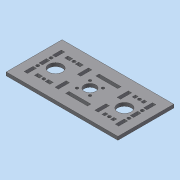
# Autodesk Inventor part: Camera-Holder_Front
Saved by Autodesk Inventor 2016 SP1 (Build 200210100, 210)
## iProperties
Created: 2016-01-24
Part Number: Camera-Holder_Front
Material: Generic
Document SubType Name: Modeling
Designer: Mohamed A.
Density: 1 g/cm^3
Appearance: Default
Author: Mohamed A.
Autodesk Inventor part; units mm, degrees
ref_plane "YZ Plane" through (0, 0, 0) normal (1, 0, 0) x (0, 1, 0)
ref_plane "XZ Plane" through (0, 0, 0) normal (0, 1, 0) x (-1, 0, 0)
ref_plane "XY Plane" through (0, 0, 0) normal (0, 0, 1) x (1, 0, 0)
sketch "Sketch1" plane through (0, 0, 0) normal (0, 0, 1) x (1, 0, 0)
  circle A0 centre (-5.816, 5.816) radius 1.25
  circle A1 centre (5.816, 5.816) radius 1.25
  circle A2 centre (5.816, -5.816) radius 1.25
  circle A3 centre (-5.816, -5.816) radius 1.25
  circle A4 centre (0, 0) radius 11
  circle A5 centre (0, 0) radius 5.125
  circle A6 centre (30.8333, 0) radius 6.096
  circle A7 centre (-30.8333, 0) radius 6.096
  line L0 (30.8333, 0) -> (-30.8333, 0) construction
  line L1 (-60, 25) -> (60, 25)
  line L2 (60, 25) -> (60, -25)
  line L3 (60, -25) -> (-60, -25)
  line L4 (-60, -25) -> (-60, 25)
  line L5 (0, 25) -> (0, -25) construction
  point P0 (0, 0)
  dimension "d9" = 2.5
  dimension "d10" = 2.5
  dimension "d11" = 2.5
  dimension "d12" = 2.5
  dimension "d33" = 120
  dimension "d34" = 50
  constraints: 12 end point, 8 centre point, 4 midpoint, 2 coincident, 2 horizontal, 2 parallel, 1 concentric, 1 perpendicular, 1 point on line, 10 other
  measures "d9" diameter of A0
  measures "d10" diameter of A1
  measures "d11" diameter of A2
  measures "d12" diameter of A3
  measures "d33" distance between parallel lines of L4 L2
  measures "d34" distance between parallel lines of L3 L1
extrude "Extrusion1" add sketch "Sketch1" along normal blind 3 contours A4 | L1 L2 L3 L4
sketch "Sketch2" plane through (0, 0, 3) normal (0, 0, 1) x (1, 0, 0)
  line L0 (42.3333, -16.6667) -> (39.3333, -16.6667)
  line L1 (39.3333, -16.6667) -> (39.3333, -8.65)
  line L2 (39.3333, -8.65) -> (42.3333, -8.65)
  line L3 (42.3333, -8.65) -> (42.3333, -16.6667)
  line L4 (39.3333, 3.35) -> (42.3333, 3.35)
  line L5 (42.3333, 3.35) -> (42.3333, -3.35)
  line L6 (42.3333, -3.35) -> (39.3333, -3.35)
  line L7 (39.3333, -3.35) -> (39.3333, 3.35)
  line L8 (42.3333, 8.65) -> (39.3333, 8.65)
  line L9 (39.3333, 8.65) -> (39.3333, 16.6667)
  line L10 (39.3333, 16.6667) -> (42.3333, 16.6667)
  line L11 (42.3333, 16.6667) -> (42.3333, 8.65)
  line L12 (-39.3333, -16.6667) -> (-42.3333, -16.6667)
  line L13 (-42.3333, -16.6667) -> (-42.3333, -8.65)
  line L14 (-42.3333, -8.65) -> (-39.3333, -8.65)
  line L15 (-39.3333, -8.65) -> (-39.3333, -16.6667)
  line L16 (-42.3333, 3.35) -> (-39.3333, 3.35)
  line L17 (-39.3333, 3.35) -> (-39.3333, -3.35)
  line L18 (-39.3333, -3.35) -> (-42.3333, -3.35)
  line L19 (-42.3333, -3.35) -> (-42.3333, 3.35)
  line L20 (-39.3333, 8.65) -> (-42.3333, 8.65)
  line L21 (-42.3333, 8.65) -> (-42.3333, 16.6667)
  line L22 (-42.3333, 16.6667) -> (-39.3333, 16.6667)
  line L23 (-39.3333, 16.6667) -> (-39.3333, 8.65)
  line L24 (19.3333, -5) -> (22.3333, -5)
  line L25 (22.3333, -5) -> (22.3333, -15)
  line L26 (22.3333, -15) -> (19.3333, -15)
  line L27 (19.3333, -15) -> (19.3333, -5)
  line L28 (22.3333, 5) -> (19.3333, 5)
  line L29 (19.3333, 5) -> (19.3333, 15)
  line L30 (19.3333, 15) -> (22.3333, 15)
  line L31 (22.3333, 15) -> (22.3333, 5)
  circle A0 centre (40.8333, 6) radius 1.4
  circle A1 centre (40.8333, -6) radius 1.4
  circle A2 centre (-40.8333, 6) radius 1.4
  circle A3 centre (-40.8333, -6) radius 1.4
  line L32 (33.4833, 12) -> (33.4833, 15)
  line L33 (33.4833, 15) -> (35.9333, 15)
  line L34 (35.9333, 15) -> (35.9333, 12)
  line L35 (35.9333, 12) -> (33.4833, 12)
  line L36 (28.1833, 15) -> (28.1833, 12)
  line L37 (28.1833, 12) -> (25.7333, 12)
  line L38 (25.7333, 12) -> (25.7333, 15)
  line L39 (25.7333, 15) -> (28.1833, 15)
  line L40 (-25.1833, 12) -> (-25.1833, 15)
  line L41 (-25.1833, 15) -> (-20.9333, 15)
  line L42 (-20.9333, 15) -> (-20.9333, 12)
  line L43 (-20.9333, 12) -> (-25.1833, 12)
  line L44 (-30.4833, 15) -> (-30.4833, 12)
  line L45 (-30.4833, 12) -> (-34.7333, 12)
  line L46 (-34.7333, 12) -> (-34.7333, 15)
  line L47 (-34.7333, 15) -> (-30.4833, 15)
  line L48 (12.8, 12) -> (-6.8, 12)
  line L49 (-6.8, 12) -> (-6.8, 15)
  line L50 (-6.8, 15) -> (12.8, 15)
  line L51 (12.8, 15) -> (12.8, 12)
  line L52 (-16.3333, -5) -> (-13.3333, -5)
  line L53 (-13.3333, -5) -> (-13.3333, -15)
  line L54 (-13.3333, -15) -> (-16.3333, -15)
  line L55 (-16.3333, -15) -> (-16.3333, -5)
  line L56 (-13.3333, 5) -> (-16.3333, 5)
  line L57 (-16.3333, 5) -> (-16.3333, 15)
  line L58 (-16.3333, 15) -> (-13.3333, 15)
  line L59 (-13.3333, 15) -> (-13.3333, 5)
  line L60 (-30.4833, -12) -> (-30.4833, -15)
  line L61 (-30.4833, -15) -> (-34.7333, -15)
  line L62 (-34.7333, -15) -> (-34.7333, -12)
  line L63 (-34.7333, -12) -> (-30.4833, -12)
  line L64 (-25.1833, -15) -> (-25.1833, -12)
  line L65 (-25.1833, -12) -> (-20.9333, -12)
  line L66 (-20.9333, -12) -> (-20.9333, -15)
  line L67 (-20.9333, -15) -> (-25.1833, -15)
  line L68 (28.1833, -12) -> (28.1833, -15)
  line L69 (28.1833, -15) -> (25.7333, -15)
  line L70 (25.7333, -15) -> (25.7333, -12)
  line L71 (25.7333, -12) -> (28.1833, -12)
  line L72 (33.4833, -15) -> (33.4833, -12)
  line L73 (33.4833, -12) -> (35.9333, -12)
  line L74 (35.9333, -12) -> (35.9333, -15)
  line L75 (35.9333, -15) -> (33.4833, -15)
  line L76 (-6.8, -12) -> (12.8, -12)
  line L77 (12.8, -12) -> (12.8, -15)
  line L78 (12.8, -15) -> (-6.8, -15)
  line L79 (-6.8, -15) -> (-6.8, -12)
  circle A4 centre (-27.8333, 13.5) radius 1.4
  circle A5 centre (-27.8333, -13.5) radius 1.4
  circle A6 centre (30.8333, -13.5) radius 1.4
  circle A7 centre (30.8333, 13.5) radius 1.4
  point P0 (0, 0)
  dimension "d35" = 2.8
  dimension "d36" = 2.8
  dimension "d37" = 5.3
  dimension "d38" = 2.65
  dimension "d39" = 2.65
  dimension "d40" = 2.8
  dimension "d41" = 2.8
  dimension "d42" = 2.65
  dimension "d43" = 2.65
  dimension "d44" = 2.8
  dimension "d45" = 5.3
  dimension "d46" = 2.65
  dimension "d47" = 2.8
  dimension "d48" = 2.8
  dimension "d49" = 5.3
  dimension "d50" = 2.65
  dimension "d51" = 2.8
  constraints: 160 end point, 40 horizontal, 40 vertical, 8 centre point, 80 other
  measures "d35" diameter of A0
  measures "d36" diameter of A1
  measures "d37" distance between parallel lines of L4 L8
  measures "d38" distance from line of A0.centre L8
  measures "d39" distance from line of L6 A1.centre
  measures "d40" diameter of A2
  measures "d41" diameter of A3
  measures "d42" distance from line of A2.centre L20
  measures "d43" distance from line of A3.centre L18
  measures "d44" diameter of A4
  measures "d45" distance between parallel lines of L44 L40
  measures "d46" distance from line of A4.centre L40
  measures "d47" diameter of A5
  measures "d48" diameter of A6
  measures "d49" distance between parallel lines of L68 L72
  measures "d50" distance from line of A6.centre L72
  measures "d51" diameter of A7
extrude "Extrusion2" cut sketch "Sketch2" against normal blind 3
equation "\"d38\" = 0.5 * d37"
equation "\"d39\" = d38"
equation "\"d42\" = d38"
equation "\"d43\" = d42"
equation "\"d46\" = 0.5 * d45"
equation "\"d50\" = 0.5 * d49"
body "Solid1"
